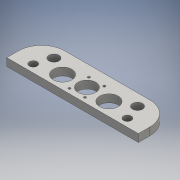
# Autodesk Inventor part: rear_plugbar
Saved by Autodesk Inventor 2016 (Build 200138000, 138)
## iProperties
Created: 2015-09-09
Part Number: rear_plugbar
Material: Generic
Document SubType Name: Modeling
Designer: oscar
Density: 1 g/cm^3
Appearance: Default
Author: oscar
Autodesk Inventor part; units mm, degrees
ref_plane "YZ Plane" through (0, 0, 0) normal (1, 0, 0) x (0, 1, 0)
ref_plane "XZ Plane" through (0, 0, 0) normal (0, 1, 0) x (-1, 0, 0)
ref_plane "XY Plane" through (0, 0, 0) normal (0, 0, 1) x (1, 0, 0)
sketch "Sketch1" plane through (0, 0, 0) normal (0, 0, 1) x (1, 0, 0)
  line L0 (170, 0) -> (0, 0)
  circle A0 centre (145.8112, 10) radius 5
  circle A1 centre (24.1888, 10) radius 5
  circle A2 centre (114.9988, 17) radius 12
  circle A3 centre (54.9988, 17) radius 12
  circle A4 centre (139, 29.91) radius 6.5
  circle A5 centre (30.9976, 29.91) radius 6.5
  arc A6 (30, 45) -> (0, 15) centre (30, 15) ccw
  arc A7 (170, 15) -> (140, 45) centre (140, 15) ccw
  circle A8 centre (84.9988, 18.5) radius 11.5
  circle A9 centre (94.9988, 6) radius 1.5
  circle A10 centre (74.9988, 31) radius 1.5
  circle A11 centre (94.9988, 31) radius 1.5
  circle A12 centre (74.9988, 6) radius 1.5
  line L1 (0, 15) -> (0, 0)
  line L2 (170, 0) -> (170, 15)
  line L3 (140, 45) -> (30, 45)
  constraints: 13 centre point, 8 end point, 4 point on circle, 1 parallel, 1 perpendicular, 1 vertical
extrude "Extrusion1" add sketch "Sketch1" along normal blind 10
body "Solid1"
